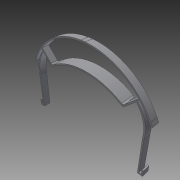
# Autodesk Inventor part: Makitronics-FaceShield
Saved by Autodesk Inventor 2015 (Build 190159000, 159)
## iProperties
Created: 2020-03-25
Part Number: Makitronics-FaceShield
Material: Generic
Document SubType Name: Modeling
Designer: Dominick Lee
Density: 1 g/cm^3
Appearance: Default
Author: Dominick Lee
Autodesk Inventor part; units mm, degrees
ref_plane "YZ Plane" through (0, 0, 0) normal (1, 0, 0) x (0, 1, 0)
ref_plane "XZ Plane" through (0, 0, 0) normal (0, 1, 0) x (-1, 0, 0)
ref_plane "XY Plane" through (0, 0, 0) normal (0, 0, 1) x (1, 0, 0)
sketch "Sketch1" plane through (0, 0, 0) normal (0, 1, 0) x (-1, 0, 0)
  arc A0 (53.7153, 50.305) -> (-53.8172, 50.3084) centre (-0.0536, -34.0093) ccw
  line L0 (73.9878, 67.2513) -> (71.8665, 65.13)
  line L1 (-74.1183, 67.2835) -> (-71.997, 65.1622)
  arc A1 (82.566, 25.5941) -> (70.4523, 63.7158) centre (32.8353, 30.777) ccw
  arc A2 (-70.5828, 63.748) -> (-82.6618, 25.6154) centre (-32.9358, 30.8434) ccw
  line L2 (82.566, 25.5941) -> (82.566, -27.4059)
  line L3 (-82.6618, 25.6154) -> (-82.6618, -27.3846)
  line L4 (-82.6618, -27.3846) -> (-89.6618, -27.3846)
  line L5 (-89.6618, -27.3846) -> (-89.6618, -18.3846)
  line L6 (82.566, -27.4059) -> (89.566, -27.4059)
  line L7 (89.566, -27.4059) -> (89.566, -18.4059)
  line L8 (-89.6618, -18.3846) -> (-87.6618, -18.3846)
  line L9 (-87.6618, -18.3846) -> (-87.6618, -25.3846)
  line L10 (-87.6618, -25.3846) -> (-84.6618, -25.3846)
  line L11 (-84.6618, -25.3846) -> (-84.6618, 25.4529)
  arc A3 (-71.997, 65.1622) -> (-84.6618, 25.4529) centre (-34.505, 31.3303) ccw
  line L12 (89.566, -18.4059) -> (87.566, -18.4059)
  line L13 (87.566, -18.4059) -> (87.566, -25.4059)
  line L14 (87.566, -25.4059) -> (84.566, -25.4059)
  line L15 (84.566, -25.4059) -> (84.566, 27.5941)
  arc A4 (84.566, 27.5941) -> (71.8665, 65.13) centre (34.2153, 31.4753) ccw
  arc A5 (91.4728, 45.0331) -> (-91.601, 45.0972) centre (-0.0799, 0.0651) ccw
  line L16 (89.2392, 45.0331) -> (91.4728, 45.0331)
  line L17 (-89.3665, 45.0972) -> (-91.601, 45.0972)
  arc A6 (53.4586, 52.8264) -> (-53.5667, 52.8259) centre (-0.0536, -34.0093) ccw
  line L18 (70.4523, 63.7158) -> (57.4497, 50.7131)
  line L19 (55.7254, 48.9889) -> (54.0544, 50.0878)
  line L20 (57.1779, 53.2834) -> (72.4501, 68.9085)
  arc A7 (89.2392, 45.0331) -> (73.9878, 67.2513) centre (-0.0799, 0.0651) ccw
  line L21 (-57.5514, 50.7166) -> (-70.5828, 63.748)
  line L22 (-55.8273, 48.9925) -> (-54.1562, 50.0913)
  line L23 (-57.2826, 53.2793) -> (-72.6098, 68.9085)
  arc A8 (72.4501, 68.9085) -> (-72.6098, 68.9085) centre (-0.0799, 0.0651) ccw
  arc A9 (-74.1183, 67.2835) -> (-89.3665, 45.0972) centre (-0.0799, 0.0651) ccw
  arc A10 (53.4586, 52.8264) -> (57.1779, 53.2834) centre (55.0325, 55.3804) ccw
  arc A11 (53.7153, 50.305) -> (57.4497, 50.7131) centre (55.3283, 52.8344) ccw
  arc A12 (-57.2826, 53.2793) -> (-53.5667, 52.8259) centre (-55.1407, 55.3798) ccw
  arc A13 (-57.5514, 50.7166) -> (-53.8172, 50.3084) centre (-55.4301, 52.838) ccw
  line L24 (-91.601, 45.0972) -> (-91.801, 45.0972)
  line L25 (-91.801, 45.0972) -> (-89.0203, 50.414)
  line L26 (-89.0203, 50.414) -> (-88.8405, 50.3199)
  line L27 (91.4728, 45.0331) -> (91.6728, 45.0331)
  line L28 (91.6728, 45.0331) -> (88.8921, 50.3498)
  line L29 (88.8921, 50.3498) -> (88.716, 50.2577)
  line L30 (0.0014, 102.0759) -> (3.0014, 102.0759)
  line L31 (0.0014, 102.0759) -> (-2.9986, 102.0759)
  line L32 (3.0014, 102.0759) -> (3.0014, 102.0186)
  line L33 (-2.9986, 102.0759) -> (-2.9986, 102.0234)
  point P0 (55.4809, 51.5472)
  point P1 (-55.5856, 51.5489)
  dimension "d5" = 178.6057
  dimension "d7" = 111.5527
  dimension "d10" = 100
  dimension "d12" = 5
  dimension "d13" = 5
  dimension "d15" = 40
  dimension "d16" = 50
  dimension "d18" = 40
  dimension "d19" = 50
  dimension "d20" = 53
  dimension "d21" = 53
  dimension "d22" = 7
  dimension "d23" = 9
  dimension "d24" = 7
  dimension "d25" = 9
  dimension "d26" = 2
  dimension "d27" = 7
  dimension "d28" = 3
  dimension "d29" = 2
  dimension "d30" = 50.5
  dimension "d31" = 2
  dimension "d32" = 2
  dimension "d33" = 7
  dimension "d34" = 3
  dimension "d35" = 53
  dimension "d36" = 50.5
  dimension "d38" = 2
  dimension "d39" = 2
  dimension "d40" = 2
  dimension "d41" = 3
  dimension "d47" = 0.2
  dimension "d48" = 6
  dimension "d49" = 62.39
  dimension "d50" = 0.2
  dimension "d51" = 6
  dimension "d52" = 62.39
  dimension "d53" = 3
  dimension "d54" = 3
  constraints: 68 end point, 38 point on circle, 14 centre point, 12 horizontal, 10 vertical, 8 tangent, 4 point on line, 3 equal radius
  measures "d5" distance of L16.start L17.start
  measures "d7" distance of L22.start L19.start
  measures "d10" radius of A0
  measures "d12" distance of L0.start L18.start
  measures "d13" distance of L1.start L21.end
  measures "d15" distance of L18.start L2.start
  measures "d16" radius of A1
  measures "d18" distance of L21.end L3.start
  measures "d19" radius of A2
  measures "d20" distance of L2.start L2.end
  measures "d21" distance of L3.start L3.end
  measures "d22" distance of L3.end L4.end
  measures "d23" distance of L4.end L5.end
  measures "d24" distance of L2.end L6.end
  measures "d25" distance of L6.end L7.end
  measures "d26" distance of L5.end L8.end
  measures "d27" distance of L8.end L9.end
  measures "d28" distance of L9.end L10.end
  measures "d29" distance of L1.end L21.end
  measures "d30" radius of A3
  measures "d31" distance of L0.end L18.start
  measures "d32" distance of L7.end L12.end
  measures "d33" distance of L12.end L13.end
  measures "d34" distance of L13.end L14.end
  measures "d35" distance of L14.end L15.end
  measures "d36" radius of A4
  measures "d38" radial gap between concentric circles of A0 A6
  measures "d39" distance of L19.start L19.end
  measures "d40" distance of L22.start L22.end
  measures "d41" radius of A10
  measures "d47" distance of L17.end L24.end
  measures "d48" distance of L24.end L25.end
  measures "d49" angle of L24 L25
  measures "d50" distance of L16.end L27.end
  measures "d51" distance of L27.end L28.end
  measures "d52" angle of L28 L27
  measures "d53" distance of L30.start L30.end
  measures "d54" distance of L30.start L31.end
extrude "Extrusion1" add sketch "Sketch1" along normal blind 10
sketch "Sketch2" plane through (0, 10, 0) normal (0, 1, 0) x (1, 0, 0)
  arc A0 (-53.4586, -52.8264) -> (-57.1779, -53.2834) centre (-55.0325, -55.3804) ccw projected
  line L0 (-57.1779, -53.2834) -> (-72.4501, -68.9085) projected
  arc A1 (-72.4501, -68.9085) -> (72.6098, -68.9085) centre (0.0799, -0.0651) ccw projected
  line L1 (72.6098, -68.9085) -> (57.2826, -53.2793) projected
  arc A2 (57.2826, -53.2793) -> (53.5667, -52.8259) centre (55.1407, -55.3798) ccw projected
  arc A3 (-53.4586, -52.8264) -> (53.5667, -52.8259) centre (0.0536, 34.0093) ccw projected
  arc A4 (-89.2392, -45.0331) -> (-73.9878, -67.2513) centre (0.0799, -0.0651) ccw projected
  line L2 (-73.9878, -67.2513) -> (-71.8665, -65.13) projected
  arc A5 (-84.566, -27.5941) -> (-71.8665, -65.13) centre (-34.2153, -31.4753) ccw projected
  line L3 (-84.566, -27.5941) -> (-84.566, 25.4059) projected
  line L4 (-84.566, 25.4059) -> (-87.566, 25.4059) projected
  line L5 (-87.566, 25.4059) -> (-87.566, 18.4059) projected
  line L6 (-87.566, 18.4059) -> (-89.566, 18.4059) projected
  line L7 (-89.566, 18.4059) -> (-89.566, 27.4059) projected
  line L8 (-89.566, 27.4059) -> (-82.566, 27.4059) projected
  line L9 (-82.566, 27.4059) -> (-82.566, -25.5941) projected
  arc A6 (-82.566, -25.5941) -> (-70.4523, -63.7158) centre (-32.8353, -30.777) ccw projected
  line L10 (-70.4523, -63.7158) -> (-57.4497, -50.7131) projected
  arc A7 (-53.7153, -50.305) -> (-57.4497, -50.7131) centre (-55.3283, -52.8344) ccw projected
  arc A8 (-53.7153, -50.305) -> (53.8172, -50.3084) centre (0.0536, 34.0093) ccw projected
  arc A9 (57.5514, -50.7166) -> (53.8172, -50.3084) centre (55.4301, -52.838) ccw projected
  line L11 (57.5514, -50.7166) -> (70.5828, -63.748) projected
  arc A10 (70.5828, -63.748) -> (82.6618, -25.6154) centre (32.9358, -30.8434) ccw projected
  line L12 (82.6618, -25.6154) -> (82.6618, 27.3846) projected
  line L13 (82.6618, 27.3846) -> (89.6618, 27.3846) projected
  line L14 (89.6618, 27.3846) -> (89.6618, 18.3846) projected
  line L15 (89.6618, 18.3846) -> (87.6618, 18.3846) projected
  line L16 (87.6618, 18.3846) -> (87.6618, 25.3846) projected
  line L17 (87.6618, 25.3846) -> (84.6618, 25.3846) projected
  line L18 (84.6618, 25.3846) -> (84.6618, -25.4529) projected
  arc A11 (71.997, -65.1622) -> (84.6618, -25.4529) centre (34.505, -31.3303) ccw projected
  line L19 (71.997, -65.1622) -> (74.1183, -67.2835) projected
  arc A12 (74.1183, -67.2835) -> (89.3665, -45.0972) centre (0.0799, -0.0651) ccw projected
  line L20 (89.3665, -45.0972) -> (91.801, -45.0972) projected
  line L21 (-91.6728, -45.0331) -> (-89.2392, -45.0331) projected
  arc A13 (-53.7153, -50.305) -> (-57.4497, -50.7131) centre (-55.3283, -52.8344) ccw projected
  line L22 (-57.4497, -50.7131) -> (-55.7058, -52.457)
  line L23 (-57.4497, -50.7131) -> (-70.4523, -63.7158) projected
  line L24 (55.8121, -52.4559) -> (57.5514, -50.7166)
  arc A14 (-88.716, -50.2577) -> (-3.0014, -102.0186) centre (0.0799, -0.0651) ccw projected
  line L25 (-88.716, -50.2577) -> (-88.8921, -50.3498) projected
  line L26 (-88.8921, -50.3498) -> (-91.6728, -45.0331) projected
  line L27 (2.9986, -102.0234) -> (2.9986, -102.0759) projected
  line L28 (2.9986, -102.0759) -> (-3.0014, -102.0759) projected
  line L29 (-3.0014, -102.0759) -> (-3.0014, -102.0186) projected
  line L30 (91.801, -45.0972) -> (89.0203, -50.414) projected
  line L31 (89.0203, -50.414) -> (88.8405, -50.3199) projected
  arc A15 (2.9986, -102.0234) -> (88.8405, -50.3199) centre (0.0799, -0.0651) ccw projected
  point P0 (0, 0)
  constraints: 4 end point, 2 point on circle, 1 perpendicular
extrude "Extrusion2" add sketch "Sketch2" along normal blind 9 contours A0 L22 A7 A8 A9 L24 A2 A3
fillet "Fillet1" radius 3 2 edges at (-56.5777, 19, 51.585) (56.6817, 19, 51.5863)
body "Solid1"
